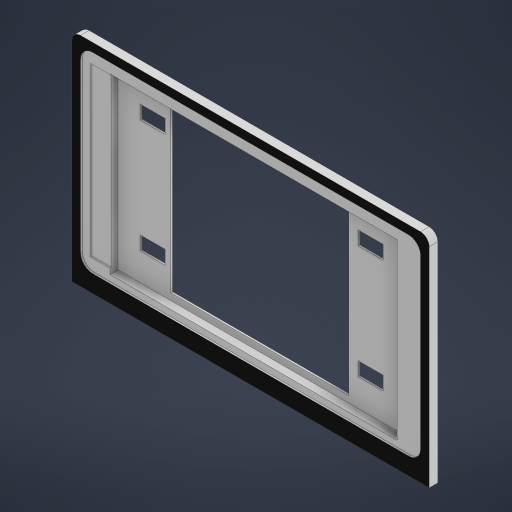
# Autodesk Inventor part: AASTRC Top case cover
Saved by Autodesk Inventor 2024.2 (Build 282272000, 272)
## iProperties
Created: 2023-07-17
Part Number: AASTRC Top case cover
Material: 일반
Document SubType Name: Modeling
Designer: wodyd
Mass: 55.8492 g
Surface Area: 390.19 cm^2
Volume: 55.8492 cm^3
Density: 1 g/cm^3
Appearance: 기본값
Author: wodyd
## iProperties of the stored document AASTRC Top case cover_3D 인쇄.ipt
Created: 2023-11-23
Part Number: AASTRC Top case cover_3D 인쇄
Material: 일반
Document SubType Name: Modeling
Designer: 6gioc
Density: 1 g/cm^3
Appearance: 기본값
Author: 6gioc
Autodesk Inventor part; units mm, degrees
ref_plane "YZ Plane" through (0, 0, 0) normal (1, 0, 0) x (0, 1, 0)
ref_plane "XZ Plane" through (0, 0, 0) normal (0, 1, 0) x (-1, 0, 0)
ref_plane "XY Plane" through (0, 0, 0) normal (0, 0, 1) x (1, 0, 0)
sketch "스케치1" plane through (0, 0, 0) normal (0, 0, 1) x (1, 0, 0)
  line L0 (-103.5, -63) -> (-103.5, 58) projected
  line L1 (-98.5, -63) -> (-103.5, -63) projected
  line L2 (-98.5, 58) -> (-98.5, -63) projected
  line L3 (98.5, 58) -> (-98.5, 58) projected
  line L4 (98.5, -63) -> (98.5, 58) projected
  line L5 (103.5, -63) -> (98.5, -63) projected
  line L6 (103.5, 58) -> (103.5, -63) projected
  arc A0 (103.5, 58) -> (98.5, 63) centre (98.5, 58) ccw projected
  line L7 (-98.5, 63) -> (98.5, 63) projected
  arc A1 (-98.5, 63) -> (-103.5, 58) centre (-98.5, 58) ccw projected
  line L8 (-98.5, -63) -> (98.5, -63)
  point P0 (0, 0)
  constraints: 2 end point, 1 collinear
extrude "돌출1" add sketch "스케치1" along normal blind 5
sketch "스케치2" plane through (0, 0, 5) normal (0, 0, 1) x (1, 0, 0)
  line L0 (-91.5, 58) -> (91.5, 58)
  line L1 (98.5, 51) -> (98.5, -46)
  line L2 (91.5, -53) -> (-91.5, -53)
  line L3 (-98.5, -46) -> (-98.5, 51)
  line L4 (98.5, 63) -> (-98.5, 63) projected
  arc A0 (-98.5, 63) -> (-103.5, 58) centre (-98.5, 58) ccw projected
  line L5 (-103.5, 58) -> (-103.5, -63) projected
  line L6 (-103.5, -63) -> (103.5, -63) projected
  line L7 (103.5, -63) -> (103.5, 58) projected
  arc A1 (103.5, 58) -> (98.5, 63) centre (98.5, 58) ccw projected
  arc A2 (-91.5, 58) -> (-98.5, 51) centre (-91.5, 51) ccw
  arc A3 (-98.5, -46) -> (-91.5, -53) centre (-91.5, -46) ccw
  arc A4 (91.5, -53) -> (98.5, -46) centre (91.5, -46) ccw
  arc A5 (98.5, 51) -> (91.5, 58) centre (91.5, 51) ccw
  point P0 (0, 0)
  point P1 (98.5, -53)
  point P2 (98.5, 58)
  point P3 (-98.5, -53)
  point P4 (0, 58)
  dimension "d2" = 197
  dimension "d3" = 111
  dimension "d4" = 207
  dimension "d5" = 126
  dimension "d6" = 103.5
  dimension "d7" = 5
  dimension "d8" = 7
  constraints: 8 end point, 8 point on circle, 8 tangent, 6 point on line, 4 centre point, 3 equal radius, 2 parallel, 1 horizontal, 1 midpoint, 1 perpendicular
  measures "d2" distance of point (98.5, -53) point (-98.5, -53)
  measures "d3" distance of point (98.5, 58) point (98.5, -53)
  measures "d4" distance between parallel lines of L7 L5
  measures "d5" distance between parallel lines of L6 L4
  measures "d6" distance from line of point (0, 58) L5
  measures "d7" distance between parallel lines of L4 L0
  measures "d8" radius of A2
extrude "돌출2" cut sketch "스케치2" against normal blind 0.9 contours L0 A5 L1 A4 L2 A3 L3 A2
sketch "스케치3" plane through (0, 0, 4.1) normal (0, 0, 1) x (1, 0, 0)
  line L0 (-82.25, 51.379) -> (83.95, 51.379)
  line L1 (83.95, 51.379) -> (83.95, -49.221)
  line L2 (83.95, -49.221) -> (-82.25, -49.221)
  line L3 (-82.25, -49.221) -> (-82.25, 51.379)
  line L4 (91.5, -53) -> (-91.5, -53) projected
  arc A0 (91.5, -53) -> (98.5, -46) centre (91.5, -46) ccw projected
  line L5 (98.5, 51) -> (98.5, -46) projected
  arc A1 (98.5, 51) -> (91.5, 58) centre (91.5, 51) ccw projected
  line L6 (-91.5, 58) -> (91.5, 58) projected
  arc A2 (-91.5, 58) -> (-98.5, 51) centre (-91.5, 51) ccw projected
  line L7 (-98.5, -46) -> (-98.5, 51) projected
  arc A3 (-98.5, -46) -> (-91.5, -53) centre (-91.5, -46) ccw projected
  point P0 (0, 0)
  dimension "d11" = 166.2
  dimension "d12" = 100.6
  dimension "d13" = 14.55
  dimension "d14" = 6.621
  constraints: 8 end point, 2 parallel, 1 horizontal, 1 perpendicular
  measures "d11" distance of L1.end L2.end
  measures "d12" distance of L0.end L1.end
  measures "d13" distance between parallel lines of L5 L1
  measures "d14" distance between parallel lines of L6 L0
sketch "스케치4" plane through (0, 0, 0) normal (0, 0, -1) x (-1, 0, 0)
  line L0 (-98.5, 63) -> (98.5, 63) projected
  arc A0 (-98.5, 63) -> (-103.5, 58) centre (-98.5, 58) ccw projected
  line L1 (-103.5, -63) -> (-103.5, 58) projected
  line L2 (103.5, -63) -> (-103.5, -63) projected
  line L3 (103.5, 58) -> (103.5, -63) projected
  arc A1 (103.5, 58) -> (98.5, 63) centre (98.5, 58) ccw projected
  line L4 (98.5, 58) -> (-98.5, 58)
  line L5 (-98.5, 58) -> (-98.5, -58)
  line L6 (-98.5, -58) -> (98.5, -58)
  line L7 (98.5, -58) -> (98.5, 58)
  point P0 (0, 0)
  dimension "d17" = 5
  constraints: 8 end point, 3 other
  measures "d17" distance between parallel lines of L0 L4
extrude "돌출4" add sketch "스케치4" along normal blind 1.303 contours L7 L6 L5 L4
extrude "돌출5" cut sketch "스케치3" against normal blind 4.403 contours L0 L1 L2 L3
sketch "스케치6" plane through (0, 0, 4.1) normal (0, 0, 1) x (1, 0, 0)
  line L0 (-93.55, 51) -> (-82.246, 51)
  line L1 (-82.246, 51) -> (-82.246, -46)
  line L2 (-82.246, -46) -> (-93.55, -46)
  line L3 (-93.55, -46) -> (-93.55, 51)
  line L4 (83.95, 51.379) -> (83.95, -49.221) projected
  line L5 (83.95, -49.221) -> (-82.25, -49.221) projected
  line L6 (-82.25, -49.221) -> (-82.25, 51.379) projected
  line L7 (-82.25, 51.379) -> (83.95, 51.379) projected
  line L8 (91.5, -53) -> (-91.5, -53) projected
  arc A0 (91.5, -53) -> (98.5, -46) centre (91.5, -46) ccw projected
  line L9 (98.5, 51) -> (98.5, -46) projected
  arc A1 (98.5, 51) -> (91.5, 58) centre (91.5, 51) ccw projected
  line L10 (-91.5, 58) -> (91.5, 58) projected
  arc A2 (-91.5, 58) -> (-98.5, 51) centre (-91.5, 51) ccw projected
  line L11 (-98.5, -46) -> (-98.5, 51) projected
  arc A3 (-98.5, -46) -> (-91.5, -53) centre (-91.5, -46) ccw projected
  point P0 (0, 0)
  point P1 (-82.25, -46)
  point P2 (-82.25, 51)
  dimension "d22" = 11.304
  dimension "d23" = 97
  dimension "d24" = 4.95
  dimension "d25" = 7
  constraints: 8 end point, 2 parallel, 1 horizontal, 1 perpendicular
  measures "d22" distance of L1.end L2.end
  measures "d23" distance of L0.end L1.end
  measures "d24" distance between parallel lines of L11 L3
  measures "d25" distance between parallel lines of L10 L0
extrude "돌출6" cut sketch "스케치6" against normal blind 0.6 contours L0 L6 L2 L3
sketch "스케치8" plane through (0, 0, -0.303) normal (0, 0, 1) x (1, 0, 0)
  line L0 (-51.5745, 50.756) -> (51.5745, 50.756)
  line L1 (51.5745, 50.756) -> (51.5745, -45.244)
  line L2 (51.5745, -45.244) -> (-51.5745, -45.244)
  line L3 (-51.5745, -45.244) -> (-51.5745, 50.756)
  line L4 (83.95, -49.221) -> (-82.25, -49.221) projected
  line L5 (83.95, 51.379) -> (83.95, -49.221) projected
  line L6 (-82.25, 51.379) -> (83.95, 51.379) projected
  line L7 (-82.25, -49.221) -> (-82.25, 51.379) projected
  arc A0 (91.5, -53) -> (98.5, -46) centre (91.5, -46) ccw projected
  line L8 (91.5, -53) -> (-91.5, -53) projected
  arc A1 (-98.5, -46) -> (-91.5, -53) centre (-91.5, -46) ccw projected
  line L9 (-98.5, -46) -> (-98.5, 51) projected
  arc A2 (-91.5, 58) -> (-98.5, 51) centre (-91.5, 51) ccw projected
  line L10 (-91.5, 58) -> (91.5, 58) projected
  arc A3 (98.5, 51) -> (91.5, 58) centre (91.5, 51) ccw projected
  line L11 (98.5, 51) -> (98.5, -46) projected
  line L12 (98.5, 63) -> (-98.5, 63) projected
  arc A4 (-98.5, 63) -> (-103.5, 58) centre (-98.5, 58) ccw projected
  line L13 (-103.5, 58) -> (-103.5, -63) projected
  line L14 (-103.5, -63) -> (103.5, -63) projected
  line L15 (103.5, -63) -> (103.5, 58) projected
  arc A5 (103.5, 58) -> (98.5, 63) centre (98.5, 58) ccw projected
  line L16 (-69.326, 40.57) -> (-54.826, 40.57)
  line L17 (-54.826, 40.57) -> (-54.826, 32.57)
  line L18 (-54.826, 32.57) -> (-69.326, 32.57)
  line L19 (-69.326, 32.57) -> (-69.326, 40.57)
  line L20 (-69.326, -25.08) -> (-54.826, -25.08)
  line L21 (-54.826, -25.08) -> (-54.826, -33.08)
  line L22 (-54.826, -33.08) -> (-69.326, -33.08)
  line L23 (-69.326, -33.08) -> (-69.326, -25.08)
  line L24 (56.95, 40.57) -> (71.45, 40.57)
  line L25 (71.45, 40.57) -> (71.45, 32.57)
  line L26 (71.45, 32.57) -> (56.95, 32.57)
  line L27 (56.95, 32.57) -> (56.95, 40.57)
  line L28 (56.95, -25.08) -> (71.45, -25.08)
  line L29 (71.45, -25.08) -> (71.45, -33.08)
  line L30 (71.45, -33.08) -> (56.95, -33.08)
  line L31 (56.95, -33.08) -> (56.95, -25.08)
  line L32 (91.5, -53) -> (-91.5, -53) projected
  arc A6 (91.5, -53) -> (98.5, -46) centre (91.5, -46) ccw projected
  line L33 (98.5, 51) -> (98.5, -46) projected
  arc A7 (98.5, 51) -> (91.5, 58) centre (91.5, 51) ccw projected
  line L34 (-91.5, 58) -> (91.5, 58) projected
  arc A8 (-91.5, 58) -> (-98.5, 51) centre (-91.5, 51) ccw projected
  line L35 (-98.5, -46) -> (-98.5, 51) projected
  arc A9 (-98.5, -46) -> (-91.5, -53) centre (-91.5, -46) ccw projected
  line L36 (-82.25, -46) -> (-93.55, -46) projected
  line L37 (-93.55, -46) -> (-93.55, 51) projected
  line L38 (-93.55, 51) -> (-82.25, 51) projected
  line L39 (-82.25, 51) -> (-82.25, 51.379) projected
  line L40 (-82.25, 51.379) -> (83.95, 51.379) projected
  line L41 (83.95, 51.379) -> (83.95, -49.221) projected
  line L42 (83.95, -49.221) -> (-82.25, -49.221) projected
  line L43 (-82.25, -49.221) -> (-82.25, -46) projected
  point P0 (0, 0)
  point P1 (0, 50.756)
  point P2 (-62.076, -25.069)
  point P3 (-61.0015, 31.581)
  point P4 (-51.5745, 2.756)
  point P5 (50.5, 51.379)
  point P6 (-50.5, 51.379)
  point P7 (-54.826, -29.08)
  point P8 (-54.826, 36.57)
  point P9 (64.2, 40.57)
  point P10 (-62.076, 40.57)
  point P11 (-69.326, -29.08)
  point P12 (-69.326, 36.57)
  dimension "d41" = 96
  dimension "d46" = 197
  dimension "d47" = 98.5
  dimension "d49" = 28.825
  dimension "d53" = 14.5
  dimension "d54" = 8
  dimension "d55" = 14.5
  dimension "d56" = 8
  dimension "d57" = 14.5
  dimension "d58" = 8
  dimension "d59" = 14.5
  dimension "d60" = 8
  dimension "d61" = 27.05
  dimension "d62" = 17.43
  dimension "d63" = 126.276
  dimension "d64" = 65.65
  constraints: 40 end point, 10 parallel, 8 midpoint, 5 horizontal, 5 perpendicular, 2 horizontal alignment, 1 point on line, 1 vertical alignment
  measures "d41" distance of L0.end L1.end
  measures "d46" distance of L12.start L12.end
  measures "d47" distance from line of L11 point (0, 50.756)
  measures "d49" vertical distance of point (-61.002, 31.581) point (-51.574, 2.756)
  measures "d53" distance of L17.end L18.end
  measures "d54" distance of L16.end L17.end
  measures "d55" distance of L21.end L22.end
  measures "d56" distance of L20.end L21.end
  measures "d57" distance of L25.end L26.end
  measures "d58" distance of L24.end L25.end
  measures "d59" distance of L29.end L30.end
  measures "d60" distance of L28.end L29.end
  measures "d61" distance between parallel lines of L11 L25
  measures "d62" distance between parallel lines of L10 L24
  measures "d63" distance of point (64.2, 40.57) point (-62.076, 40.57)
  measures "d64" distance of point (-69.326, -29.08) point (-69.326, 36.57)
extrude "돌출8" cut sketch "스케치8" against normal blind 2.5 contours L0 L1 L2 L3 | L16 L17 L18 L19 | L20 L21 L22 L23 | L24 L25 L26 L27 | L28 L29 L30 L31
